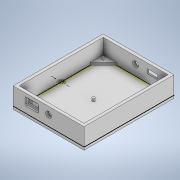
# Autodesk Inventor part: WIP
Saved by Autodesk Inventor 2021 (Build 250183000, 183)
## iProperties
Created: 2021-04-28
Part Number: WIP
Material: Generic
Document SubType Name: Modeling
Designer: mista
Density: 1 g/cm^3
Appearance: Default
Author: mista
Autodesk Inventor part; units mm, degrees
ref_plane "YZ Plane" through (0, 0, 0) normal (1, 0, 0) x (0, 1, 0)
ref_plane "XZ Plane" through (0, 0, 0) normal (0, 1, 0) x (-1, 0, 0)
ref_plane "XY Plane" through (0, 0, 0) normal (0, 0, 1) x (1, 0, 0)
sketch "Sketch1" plane through (0, 0, 0) normal (0, 1, 0) x (-1, 0, 0)
  line L0 (0, 0) -> (54.0004, 0)
  line L1 (54.0004, 0) -> (54.0004, -70.6374)
  line L2 (54.0004, -70.6374) -> (0, -70.6374)
  line L3 (0, -70.6374) -> (0, 0)
  circle A0 centre (51.9049, -68.5419) radius 1.0795
  circle A1 centre (3.3909, -67.8053) radius 1.0795
  circle A2 centre (51.9049, -1.8923) radius 1.0795
  circle A3 centre (1.7674, -2.3495) radius 1.0795
  dimension "d0" = 54.0004
  dimension "d1" = 70.6374
  dimension "d2" = 2.159
  dimension "d6" = 1.016
  dimension "d8" = 1.016
  dimension "d11" = 2.159
  dimension "d12" = 48.514
  dimension "d13" = 1.7526
  dimension "d15" = 66.6496
  dimension "d16" = 2.159
  dimension "d17" = 1.016
  dimension "d18" = 2.159
  dimension "d20" = 65.4558
  dimension "d21" = 50.1375
  constraints: 8 end point, 4 centre point, 2 parallel, 1 horizontal, 1 perpendicular
  measures "d0" distance of L1.end L2.end
  measures "d1" distance of L0.end L1.end
  measures "d2" diameter of A0
  measures "d6" distance edge to line of A0 L2
  measures "d8" distance edge to line of A0 L1
  measures "d11" diameter of A1
  measures "d12" horizontal distance of A1.centre A0.centre
  measures "d13" distance edge to line of A1 L2
  measures "d15" distance of A0.centre A2.centre
  measures "d16" diameter of A2
  measures "d17" distance edge to line of A2 L1
  measures "d18" diameter of A3
  measures "d20" vertical distance of A1.centre A3.centre
  measures "d21" horizontal distance of A3.centre A2.centre
sketch "Sketch2" plane through (0, 0, 0) normal (0, 1, 0) x (-1, 0, 0)
  line L0 (54.0004, 0) -> (54.0004, -70.6374) projected
  line L1 (0, 0) -> (54.0004, 0) projected
  line L2 (0, -70.6374) -> (0, 0) projected
  line L3 (54.0004, -70.6374) -> (0, -70.6374) projected
  line L4 (55.2704, -71.9074) -> (55.2704, 1.27)
  line L5 (55.2704, 1.27) -> (-1.27, 1.27)
  line L6 (-1.27, 1.27) -> (-1.27, -71.9074)
  line L7 (-1.27, -71.9074) -> (55.2704, -71.9074)
  line L8 (57.8104, 3.81) -> (57.8104, -74.4474)
  line L9 (57.8104, -74.4474) -> (-3.81, -74.4474)
  line L10 (-3.81, -74.4474) -> (-3.81, 3.81)
  line L11 (-3.81, 3.81) -> (57.8104, 3.81)
  dimension "d22" = 1.27
  dimension "d23" = 2.54
  constraints: 16 end point, 6 other
  measures "d22" distance between parallel lines of L0 L4
  measures "d23" distance between parallel lines of L4 L8
extrude "Extrusion1" add sketch "Sketch2" against normal blind 2.54 contours L0 L3 L2 L1 | L7 L6 L5 L4 | L8 L9 L10 L11
extrude "Extrusion2" add sketch "Sketch2" along normal blind 15.24 contours L8 L9 L10 L11
sketch "Sketch3" plane through (0, 0, 0) normal (0, 1, 0) x (1, 0, 0)
  line L0 (-55.2704, 71.9074) -> (-55.2704, -1.27) projected
  line L1 (-55.2704, -1.27) -> (1.27, -1.27) projected
  line L2 (1.27, -1.27) -> (1.27, 71.9074) projected
  line L3 (1.27, 71.9074) -> (-55.2704, 71.9074) projected
  line L4 (1.27, 10.16) -> (-10.16, -1.27)
  line L5 (-0.6357, 8.2543) -> (6.4192, 8.2543) construction
  line L6 (1.27, -1.27) -> (-55.2704, -1.27) construction
  line L7 (-27.0002, -1.27) -> (-27.0002, 8.9046) construction
  line L8 (1.27, 71.9074) -> (1.27, -1.27) construction
  line L9 (1.27, 35.3187) -> (-18.2366, 35.3187) construction
  line L10 (-55.2704, 10.16) -> (-43.8404, -1.27)
  line L11 (1.27, 60.4774) -> (-10.16, 71.9074)
  line L12 (-55.2704, 60.4774) -> (-43.8404, 71.9074)
  point P0 (0, 0)
  point P1 (-10.16, 71.9074)
  point P2 (1.27, 60.4774)
  point P3 (-55.2704, 60.4774)
  point P4 (-43.8404, 71.9074)
  dimension "d28" = 135
  dimension "d29" = 11.43
  constraints: 14 end point, 6 symmetric about line, 3 point on line, 2 horizontal, 2 midpoint, 1 vertical
  measures "d28" angle of L4 L5
  measures "d29" horizontal distance of L4.start L4.end
extrude "Extrusion3" add sketch "Sketch3" along normal blind 2.032 contours L3 L12 L0 | L10 L1 L0 | L3 L2 L11 | L4 L2 L1
extrude "Extrusion4" add sketch "Sketch1" along normal blind 3.81 contours A0 | A1 | A2 | A3
thicken "Thicken1" operation add thickness 0.127 both sides no extend neighbours yes toward (0.8451901, 0, -0.5344658) faces at (-4.3033, 3.2173, -67.2283)
thicken "Thicken2" operation add thickness 0.127 both sides no extend neighbours yes toward (0.9870503, 0, -0.1604113) faces at (-2.8329, 3.2173, -2.1763)
thicken "Thicken3" operation add thickness 0.127 both sides no extend neighbours yes toward (-0.6324454, 0, -0.774605) faces at (-51.2222, 3.2173, -1.0561)
thicken "Thicken4" operation add thickness 0.127 both sides no extend neighbours yes toward (-0.8451901, 0, 0.5344658) faces at (-50.9925, 2.6247, -69.1189)
sketch "Sketch5" plane through (-57.8104, -2.54, 3.81) normal (0, 0, 1) x (1, 0, 0)
  line L0 (0, 0) -> (0, 17.78) projected
  line L1 (61.6204, 0) -> (0, 0) projected
  line L2 (61.6204, 17.78) -> (61.6204, 0) projected
  line L3 (0, 17.78) -> (61.6204, 17.78) projected
  line L4 (13.97, 2.54) -> (13.97, 4.572) projected
  line L5 (13.97, 4.572) -> (2.54, 4.572) projected
  line L6 (2.54, 4.572) -> (2.54, 17.78) projected
  line L7 (59.0804, 17.78) -> (2.54, 17.78) projected
  line L8 (59.0804, 4.572) -> (59.0804, 17.78) projected
  line L9 (59.0804, 4.572) -> (47.6504, 4.572) projected
  line L10 (47.6504, 4.572) -> (47.6504, 2.54) projected
  line L11 (13.97, 2.54) -> (47.6504, 2.54) projected
  line L12 (57.8104, 2.54) -> (3.81, 2.54) projected
  line L13 (3.81, 2.54) -> (3.81, 17.78) construction
  line L14 (0, 17.78) -> (61.6204, 17.78) construction
  line L15 (57.8104, 2.54) -> (57.8104, 17.78) construction
  line L16 (11.7348, 13.4112) -> (20.6248, 13.4112)
  line L17 (20.6248, 13.4112) -> (20.6248, 9.6012)
  line L18 (20.6248, 9.6012) -> (11.7348, 9.6012)
  line L19 (11.7348, 9.6012) -> (11.7348, 13.4112)
  line L20 (16.1798, 13.4112) -> (16.1798, 9.6012) construction
  line L21 (11.7348, 11.5062) -> (20.6248, 11.5062) construction
  dimension "d70" = 8.89
  dimension "d71" = 3.81
  dimension "d73" = 12.3698
  dimension "d74" = 6.9342
  constraints: 16 end point, 4 midpoint, 3 parallel, 2 perpendicular, 2 point on line, 1 horizontal
  measures "d70" distance of L17.end L18.end
  measures "d71" distance of L16.end L17.end
  measures "d73" distance between parallel lines of L13 L20
  measures "d74" distance between parallel lines of L5 L21
extrude "Extrusion5" cut sketch "Sketch5" against normal blind 2.54 contours L16 L17 L18 L19
sketch "Sketch6" plane through (-57.8104, -2.54, 3.81) normal (0, 0, 1) x (1, 0, 0)
  line L0 (20.6248, 13.4112) -> (20.6248, 9.6012) projected
  line L1 (20.6248, 9.6012) -> (11.7348, 9.6012) projected
  line L2 (11.7348, 9.6012) -> (11.7348, 13.4112) projected
  line L3 (11.7348, 13.4112) -> (20.6248, 13.4112) projected
  line L4 (0, 0) -> (0, 17.78) projected
  line L5 (61.6204, 0) -> (0, 0) projected
  line L6 (61.6204, 17.78) -> (61.6204, 0) projected
  line L7 (0, 17.78) -> (61.6204, 17.78) projected
  line L8 (22.1488, 13.9192) -> (22.1488, 9.0932)
  line L9 (21.1328, 8.0772) -> (11.2268, 8.0772)
  line L10 (10.2108, 9.0932) -> (10.2108, 13.9192)
  line L11 (11.2268, 14.9352) -> (21.1328, 14.9352)
  arc A0 (11.2268, 14.9352) -> (10.2108, 13.9192) centre (11.2268, 13.9192) ccw
  arc A1 (22.1488, 13.9192) -> (21.1328, 14.9352) centre (21.1328, 13.9192) ccw
  arc A2 (21.1328, 8.0772) -> (22.1488, 9.0932) centre (21.1328, 9.0932) ccw
  arc A3 (10.2108, 9.0932) -> (11.2268, 8.0772) centre (11.2268, 9.0932) ccw
  point P0 (57.8104, 2.54)
  dimension "d78" = 6.858
  dimension "d79" = 1.016
  constraints: 8 end point, 8 point on circle, 8 tangent, 4 centre point, 3 equal radius, 3 other
  measures "d78" distance between parallel lines of L9 L11
  measures "d79" radius of A0
extrude "Extrusion6" cut sketch "Sketch6" against normal blind 1.27 contours L8 A2 L9 A3 L10 A0 L11 A1
sketch "Sketch7" plane through (-57.8104, -2.54, 3.81) normal (0, 0, 1) x (1, 0, 0)
  line L0 (20.6248, 9.6012) -> (20.6248, 13.4112) projected
  line L1 (20.6248, 13.4112) -> (11.7348, 13.4112) projected
  line L2 (11.7348, 13.4112) -> (11.7348, 9.6012) projected
  line L3 (11.7348, 9.6012) -> (20.6248, 9.6012) projected
  line L4 (13.97, 2.54) -> (13.97, 4.572) projected
  line L5 (13.97, 4.572) -> (2.54, 4.572) projected
  line L6 (2.54, 4.572) -> (2.54, 17.78) projected
  line L7 (59.0804, 17.78) -> (2.54, 17.78) projected
  line L8 (59.0804, 4.572) -> (59.0804, 17.78) projected
  line L9 (59.0804, 4.572) -> (47.6504, 4.572) projected
  line L10 (47.6504, 4.572) -> (47.6504, 2.54) projected
  line L11 (13.97, 2.54) -> (47.6504, 2.54) projected
  line L12 (57.8104, 2.54) -> (3.81, 2.54) projected
  circle A0 centre (30.8102, 11.5062) radius 2.54
  line L13 (20.6248, 9.6012) -> (20.6248, 13.4112) construction
  line L14 (20.6248, 11.5062) -> (40.0653, 11.5062) construction
  dimension "d82" = 5.08
  dimension "d84" = 0
  constraints: 2 end point, 1 centre point, 1 horizontal, 1 midpoint
  measures "d82" diameter of A0
  measures "d84" distance from line of L14 A0.centre
extrude "Extrusion7" cut sketch "Sketch7" against normal blind 2.54 contours A0
sketch "Sketch9" plane through (0, 0, 0) normal (0, 1, 0) x (1, 0, 0)
  line L0 (3.81, -3.81) -> (-57.8104, -3.81) projected
  line L1 (-27.0002, -3.81) -> (-27.0002, 74.4474) construction
  line L2 (3.81, 74.4474) -> (-57.8104, 74.4474) projected
  line L3 (3.81, 74.4474) -> (3.81, -3.81) projected
  line L4 (3.81, 35.3187) -> (-27.0002, 35.3187) construction
  circle A0 centre (-27.0002, 35.3187) radius 1.27
  point P0 (0, 0)
  dimension "d87" = 2.54
  constraints: 4 end point, 4 midpoint, 1 centre point, 1 coincident
  measures "d87" diameter of A0
extrude "Extrusion8" add sketch "Sketch9" along normal blind 2.032
pattern_circular "Circular Pattern1" count 2 over 360 about axis through (-27.0002, 0, -35.3187) along (0, 1, 0) of "Extrusion7", "Extrusion5", "Extrusion6"
body "Solid1"
